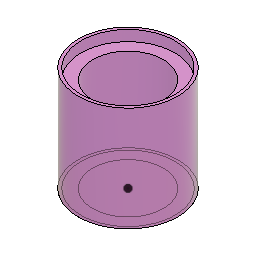
3_8 inch X-axis Bushing Holder v22 (Autodesk Fusion 360 design; units mm, degrees)
Autodesk Fusion 360 part; units mm, degrees
note: some values were not read from the file. Set by a fixed rule: which sketch regions a step uses.
sketch "Sketch1" plane through (0, 0, 0) normal (0, 0, 1) x (1, 0, 0) in component "Holder V1"
  circle A0 centre (0, 0) radius 6.325
  line L0 (0, 0) -> (-10.0178, 0) construction
  line L1 (-10.0178, -2.5) -> (-10.0178, 2.5) construction
  line L2 (-10.0178, 2.5) -> (-15.0178, 2.5)
  line L3 (-15.0178, 2.5) -> (-15.0178, -2.5)
  line L4 (-15.0178, -2.5) -> (-10.0178, -2.5)
  arc A1 (-10.0178, 2.5) -> (-10.0178, -2.5) centre (0, 0) ccw construction
  line L5 (-2.5, -10.0178) -> (-2.5, -15.0178)
  line L6 (-2.5, -15.0178) -> (2.5, -15.0178)
  line L7 (2.5, -15.0178) -> (2.5, -10.0178)
  line L8 (10.0178, -2.5) -> (15.0178, -2.5)
  line L9 (15.0178, -2.5) -> (15.0178, 2.5)
  line L10 (15.0178, 2.5) -> (10.0178, 2.5)
  line L11 (2.5, 10.0178) -> (2.5, 15.0178)
  line L12 (2.5, 15.0178) -> (-2.5, 15.0178)
  line L13 (-2.5, 15.0178) -> (-2.5, 10.0178)
  arc A2 (-10.0178, -2.5) -> (-2.5, -10.0178) centre (0, 0) ccw
  arc A3 (-2.5, -10.0178) -> (2.5, -10.0178) centre (0, 0) ccw construction
  arc A4 (2.5, -10.0178) -> (10.0178, -2.5) centre (0, 0) ccw
  arc A5 (10.0178, -2.5) -> (10.0178, 2.5) centre (0, 0) ccw construction
  arc A6 (10.0178, 2.5) -> (2.5, 10.0178) centre (0, 0) ccw
  arc A7 (-2.5, 10.0178) -> (-10.0178, 2.5) centre (0, 0) ccw
  arc A8 (2.5, 10.0178) -> (-2.5, 10.0178) centre (0, 0) ccw construction
  dimension "d13" = 12.65
  dimension "d14" = 5
  dimension "d15" = 20.65
  dimension "d17" = 360
  measures "d13" diameter of A0
  measures "d15" diameter of A2
extrude "Extrude1" add sketch "Sketch1" along normal blind 15.8 makes body 1 in component "Holder V1"
chamfer "Chamfer1" distance 1 angle 60 1 edges at (-5.897, 2.2872, 15.8) measured on face at (0.8333, -13.3511, 15.8) on bodies 1 in component "Holder V1"
sketch "Sketch1 (2)" plane through (0, 0, 0) normal (0, 0, 1) x (1, 0, 0) in component "Holder V2.3"
  arc A0 (-2.5, 10.0178) -> (-10.0178, 2.5) centre (0, 0) ccw construction
  line L0 (-10.0178, 2.5) -> (-15.0178, 2.5)
  line L1 (-15.0178, 2.5) -> (-15.0178, -2.5)
  line L2 (-15.0178, -2.5) -> (-10.0178, -2.5)
  arc A1 (-10.0178, -2.5) -> (-2.5, -10.0178) centre (0, 0) ccw
  line L3 (-2.5, -10.0178) -> (-2.5, -15.0178)
  line L4 (-2.5, -15.0178) -> (2.5, -15.0178)
  line L5 (2.5, -15.0178) -> (2.5, -10.0178)
  arc A2 (2.5, -10.0178) -> (10.0178, -2.5) centre (0, 0) ccw
  line L6 (10.0178, -2.5) -> (15.0178, -2.5)
  line L7 (15.0178, -2.5) -> (15.0178, 2.5)
  line L8 (15.0178, 2.5) -> (10.0178, 2.5)
  arc A3 (10.0178, 2.5) -> (2.5, 10.0178) centre (0, 0) ccw
  line L9 (2.5, 10.0178) -> (2.5, 15.0178)
  line L10 (2.5, 15.0178) -> (-2.5, 15.0178)
  line L11 (-2.5, 15.0178) -> (-2.5, 10.0178)
  circle A4 centre (0, 0) radius 7.325 construction
  line L12 (-14.0178, 1.5) -> (-14.0178, -1.5)
  line L13 (-14.0178, -1.5) -> (-9.2036, -1.5)
  arc A5 (-9.2036, -1.5) -> (-1.5, -9.2036) centre (0, 0) ccw
  line L14 (-1.5, -9.2036) -> (-1.5, -14.0178)
  line L15 (-1.5, -14.0178) -> (1.5, -14.0178)
  line L16 (1.5, -14.0178) -> (1.5, -9.2036)
  arc A6 (1.5, -9.2036) -> (9.2036, -1.5) centre (0, 0) ccw
  line L17 (9.2036, -1.5) -> (14.0178, -1.5)
  line L18 (14.0178, -1.5) -> (14.0178, 1.5)
  line L19 (14.0178, 1.5) -> (9.2036, 1.5)
  arc A7 (9.2036, 1.5) -> (1.5, 9.2036) centre (0, 0) ccw
  line L20 (1.5, 9.2036) -> (1.5, 14.0178)
  line L21 (1.5, 14.0178) -> (-1.5, 14.0178)
  line L22 (-1.5, 14.0178) -> (-1.5, 9.2036)
  arc A8 (-1.5, 9.2036) -> (-9.2036, 1.5) centre (0, 0) ccw
  line L23 (-9.2036, 1.5) -> (-14.0178, 1.5)
  circle A9 centre (0, 0) radius 6.325 construction
  circle A10 centre (0, 0) radius 6.3251
  dimension "d22" = 1
  dimension "d28" = 0.0001
  measures "d22" distance of L1
extrude "Extrude1'" add sketch "Sketch1 (2)" along normal blind 20 separate body makes body 2 in component "Holder V2.3"
sketch "Sketch1 (3)" plane through (0, 0, 0) normal (0, 0, 1) x (1, 0, 0) in component "Holder V3.1"
  circle A0 centre (0, 0) radius 5
  circle A1 centre (0, 0) radius 6.4 construction
  line L0 (0, 0) -> (-9.4, 0) construction
  line L1 (-9.1848, 0) -> (-9.1848, 2) construction
  line L2 (-9.1848, 2) -> (-17.1959, 2)
  line L3 (-17.1959, 2) -> (-17.1959, -2)
  line L4 (-17.1959, -2) -> (-9.1848, -2)
  line L5 (-9.1848, -2) -> (-9.1848, 0) construction
  arc A2 (-9.4, 0) -> (-9.1848, -2) centre (0, 0) ccw construction
  arc A3 (-9.1848, 2) -> (-9.4, 0) centre (0, 0) ccw construction
  line L6 (-2, -9.1848) -> (-2, -17.1959)
  line L7 (-2, -17.1959) -> (2, -17.1959)
  line L8 (2, -17.1959) -> (2, -9.1848)
  line L9 (9.1848, -2) -> (17.1959, -2)
  line L10 (17.1959, -2) -> (17.1959, 2)
  line L11 (17.1959, 2) -> (9.1848, 2)
  line L12 (2, 9.1848) -> (2, 17.1959)
  line L13 (2, 17.1959) -> (-2, 17.1959)
  line L14 (-2, 17.1959) -> (-2, 9.1848)
  arc A4 (9.1848, -2) -> (9.1848, 2) centre (0, 0) ccw construction
  arc A5 (9.1848, 2) -> (2, 9.1848) centre (0, 0) ccw
  arc A6 (-2, 9.1848) -> (-9.1848, 2) centre (0, 0) ccw
  arc A7 (-9.1848, -2) -> (-2, -9.1848) centre (0, 0) ccw
  arc A8 (2, -9.1848) -> (9.1848, -2) centre (0, 0) ccw
  arc A9 (-2, -9.1848) -> (2, -9.1848) centre (0, 0) ccw construction
  arc A10 (2, 9.1848) -> (-2, 9.1848) centre (0, 0) ccw construction
  dimension "d29" = 18.8
  dimension "d30" = 12.8
  dimension "d31" = 10
  dimension "d32" = 4
  dimension "d34" = 360
  measures "d29" diameter of A7
  measures "d30" diameter of A1
  measures "d31" diameter of A0
extrude "Extrude1''" add sketch "Sketch1 (3)" along normal blind 16 separate body makes body 3 in component "Holder V3.1"
chamfer "Chamfer1'" distance 1 angle 45 1 edges at (-4.6616, 1.8081, 16) on bodies 3 in component "Holder V3.1"
fillet "Fillet1" radius 1.5 32 edges at (6.6468, 6.6468, 16) (2, 13.1903, 16) (0, 17.1959, 16) (-2, 13.1903, 16) (-6.6468, 6.6468, 16) (-13.1903, 2, 16) (-17.1959, 0, 16) (-13.1903, -2, 16) (-6.6468, -6.6468, 16) (-2, -13.1903, 16) (0, -17.1959, 16) (2, -13.1903, 16) (6.6468, -6.6468, 16) (13.1903, -2, 16) (17.1959, 0, 16) (13.1903, 2, 16) (17.1959, 0, 0) (13.1903, 2, 0) (6.6468, 6.6468, 0) (2, 13.1903, 0) (-2, 13.1903, 0) (0, 17.1959, 0) (-6.6468, 6.6468, 0) (-13.1903, 2, 0) (-17.1959, 0, 0) (-13.1903, -2, 0) (-2, -13.1903, 0) (0, -17.1959, 0) (2, -13.1903, 0) (6.6468, -6.6468, 0) (13.1903, -2, 0) (-6.6468, -6.6468, 0) on bodies 3 in component "Holder V3.1"
sketch "Sketch1 (4)" plane through (0, 0, 0) normal (0, 1, 0) x (1, 0, 0) in component "Holder Test V4.2"
  circle A0 centre (0, 0) radius 6.3
  circle A1 centre (0, 0) radius 7.8
  circle A2 centre (16, 0) radius 6.4
  circle A3 centre (16, 0) radius 7.9
  circle A4 centre (32, 0) radius 6.5
  circle A5 centre (32, 0) radius 8
  circle A6 centre (0, 16) radius 6.8
  circle A7 centre (0, 16) radius 8.3
  circle A8 centre (16, 16) radius 6.7
  circle A9 centre (16, 16) radius 8.2
  circle A10 centre (32, 16) radius 6.6
  circle A11 centre (32, 16) radius 8.1
  line L0 (-0.5169, -7.65) -> (0.3, -7.65) construction
  line L1 (0.3, -7.65) -> (0.3, -5.9) construction
  line L2 (0.3, -5.9) -> (-0.5169, -5.9) construction
  line L3 (-0.5169, -5.9) -> (-0.5169, -7.65) construction
  line L4 (15.5931, -7.9846) -> (16.0546, -7.9846) construction
  line L5 (16.0546, -7.9846) -> (16.0546, -6.2346) construction
  line L6 (16.0546, -6.2346) -> (15.5931, -6.2346) construction
  line L7 (15.5931, -6.2346) -> (15.5931, -7.9846) construction
  line L8 (31.4703, -7.85) -> (32.3, -7.85) construction
  line L9 (32.3, -7.85) -> (32.3, -6.1) construction
  line L10 (32.3, -6.1) -> (31.4703, -6.1) construction
  line L11 (31.4703, -6.1) -> (31.4703, -7.85) construction
  line L12 (31.4797, 22.7) -> (32.3, 22.7) construction
  line L13 (32.3, 22.7) -> (32.3, 24.45) construction
  line L14 (32.3, 24.45) -> (31.4797, 24.45) construction
  line L15 (31.4797, 24.45) -> (31.4797, 22.7) construction
  line L16 (15.3335, 22.8) -> (16.2, 22.8) construction
  line L17 (16.2, 22.8) -> (16.2, 24.55) construction
  line L18 (16.2, 24.55) -> (15.3335, 24.55) construction
  line L19 (15.3335, 24.55) -> (15.3335, 22.8) construction
  line L20 (-0.6, 22.9) -> (0.2306, 22.9) construction
  line L21 (0.2306, 22.9) -> (0.2306, 24.65) construction
  line L22 (0.2306, 24.65) -> (-0.6, 24.65) construction
  line L23 (-0.6, 24.65) -> (-0.6, 22.9) construction
  line L24 (0, 0) -> (32, 0)
  line L25 (32, 0) -> (32, 16)
  line L26 (32, 16) -> (0, 16)
  line L27 (0, 16) -> (0, 0)
  line L28 (0, 16) -> (0, 17.5)
  line L29 (0, 17.5) -> (32, 17.5)
  line L30 (32, 17.5) -> (32, 16)
  line L31 (32, 0) -> (32, -1.5)
  line L32 (32, -1.5) -> (0, -1.5)
  line L33 (0, -1.5) -> (0, 0)
  line L34 (0, -1.5) -> (-1.5, -1.5)
  line L35 (-1.5, -1.5) -> (-1.5, 17.5)
  line L36 (-1.5, 17.5) -> (0, 17.5)
  line L37 (32, 17.5) -> (33.5, 17.5)
  line L38 (33.5, 17.5) -> (33.5, -1.5)
  line L39 (33.5, -1.5) -> (32, -1.5)
  line L40 (-1.5, 0) -> (32, 17.5)
  line L41 (0, -1.5) -> (33.5, 16)
  line L42 (32, 0) -> (33.5, 0)
  line L43 (33.5, 0) -> (0, 17.5)
  line L44 (32, -1.5) -> (-1.5, 16)
  line L45 (-1.5, 0) -> (-7.8, 0) construction
  line L46 (-7.8, 0) -> (-10.3, 0)
  line L47 (-10.3, 0) -> (-10.3, -2.5)
  line L48 (-10.3, -2.5) -> (-7.3885, -2.5)
  dimension "d40" = 12.6
  dimension "d41" = 15.6
  dimension "d46" = 12.8
  dimension "d47" = 13
  dimension "d48" = 13.2
  dimension "d49" = 13.4
  dimension "d50" = 13.6
  dimension "d51" = 15.8
  dimension "d52" = 16
  dimension "d53" = 16.2
  dimension "d54" = 16.4
  dimension "d55" = 16.6
  dimension "d61" = 2.5
  dimension "d62" = 2.5
  measures "d40" diameter of A0
  measures "d41" diameter of A1
  measures "d46" diameter of A2
  measures "d47" diameter of A4
  measures "d48" diameter of A10
  measures "d49" diameter of A8
  measures "d50" diameter of A6
  measures "d51" diameter of A3
  measures "d52" diameter of A5
  measures "d53" diameter of A11
  measures "d54" diameter of A9
  measures "d55" diameter of A7
extrude "Extrude1'''" add sketch "Sketch1 (4)" along normal blind 5 separate body contours A0 A1 L24 L32 | A0 A1 L24 L41 | A0 A1 L40 L41 | A0 A1 L32 L35 | A1 A3 L24 L32 | A0 A1 A7 L27 L40 | A1 A3 L40 L41 L44 | A0 A1 A7 L27 L35 | A2 A3 L24 L32 | A2 A3 L24 L41 | A2 A3 L41 L44 | A1 A7 L35 | A1 L46 L47 L48 | A2 A3 L32 | A1 A7 L27 | A1 A7 L27 | A1 A6 A7 L27 L44 | A9 L40 L44 | A3 A9 L40 L44 | A3 A9 L41 L44 | A1 A6 A7 L27 L35 | A6 A7 A9 L29 L35 | A2 A3 L24 L32 | A3 A5 L24 L32 | A2 A3 L24 L44 | A6 A7 L43 L44 | A7 A9 L43 L44 | A3 A9 L40 L43 | A8 A9 L40 L43 L44 | A9 L44 | A3 A9 | A2 L41 L44 | A2 A3 L41 L44 | A7 A8 A9 A11 L29 | A7 A9 L29 | A4 A5 L32 L38 | A4 A5 L24 L32 | A6 A7 A9 L26 L43 | A8 L40 L43 | A8 A9 L40 L41 L43 | A3 A9 L41 L43 | A3 A5 L41 L43 L44 | A7 A8 L26 L29 | A7 A9 L26 L29 | A9 A10 A11 L29 L38 | A9 A11 L29 | A6 A9 L26 L29 | A4 A5 L24 L44 | A7 A9 L26 | A7 A8 A9 L26 L43 | A9 L41 L43 | A9 A10 L26 L29 | A9 A11 L26 L29 | A8 A11 L26 L29 | A4 A5 L43 L44 | A4 A5 A11 L25 L38 | A5 A11 L38 | A8 A9 A11 L26 L40 | A9 L41 | A4 A5 A11 L25 L43 | A9 A10 A11 L26 L40 | A9 A11 L26 | A5 A10 A11 L25 L38 | A5 A11 L25 | A9 A11 L40 L41 | A5 A10 A11 L25 L41 | A5 A11 L25 | A10 A11 L40 L41 makes body 4 in component "Holder Test V4.2"
sketch "Sketch1 (5)" plane through (0, 0, 0) normal (0, 1, 0) x (1, 0, 0) in component "Holder V4.2"
  circle A0 centre (0, 0) radius 6.7
  circle A1 centre (0, 0) radius 9.45
  dimension "d63" = 13.4
  dimension "d64" = 18.9
  measures "d63" diameter of A0
  measures "d64" diameter of A1
extrude "Extrude1''''" add sketch "Sketch1 (5)" along normal blind 16 separate body makes body 5 in component "Holder V4.2"
sketch "Sketch1 (6)" plane through (0, 0, 0) normal (0, 1, 0) x (1, 0, 0) in component "Holder (for bronze 1/2in OD bushings) V5"
  circle A0 centre (0, 0) radius 6.65
  circle A1 centre (0, 0) radius 9.4
  circle A2 centre (0, 0) radius 8.8562
  dimension "d63_1" = 13.3
  dimension "d64_1" = 18.8
  dimension "d67" = 17.7125
  measures "d63_1" diameter of A0
  measures "d64_1" diameter of A1
  measures "d67" diameter of A2
extrude "Extrude1'''''" add sketch "Sketch1 (6)" along normal blind 17.8 separate body contours A1 | A2 makes body 6 in component "Holder (for bronze 1/2in OD bushings) V5"
extrude "Extrude2" add sketch "Sketch1 (6)" along normal blind 2 from surface at 17.8 contours A1 bodies 6 in component "Holder (for bronze 1/2in OD bushings) V5"
component "Holder V1" placed x (1, 0, 0) y (0, 1, 0) z (0, 0, 1) at (0, 0, 0)
component "Holder V2.3" placed x (1, 0, 0) y (0, 1, 0) z (0, 0, 1) at (0, 0, 0)
component "Holder V3.1" placed x (1, 0, 0) y (0, 1, 0) z (0, 0, 1) at (0, 0, 0)
component "Holder Test V4.2" placed x (1, 0, 0) y (0, 1, 0) z (0, 0, 1) at (0, 0, 0)
component "Holder V4.2" placed x (1, 0, 0) y (0, 1, 0) z (0, 0, 1) at (0, 0, 0)
component "Holder (for bronze 1/2in OD bushings) V5" placed x (1, 0, 0) y (0, 1, 0) z (0, 0, 1) at (0, 0, 0)
equation "d15 = d13 + ( ( 2 * 4 ) * 1 mm )"
equation "d29 = d30 + ( ( 3 * 2 ) * 1 mm )"
equation "d41 = d40 + 3 mm"
equation "d46 = d40 + 0.2 mm"
equation "d47 = d46 + 0.2 mm"
equation "d48 = d47 + 0.2 mm"
equation "d49 = d48 + 0.2 mm"
equation "d50 = d49 + 0.2 mm"
equation "d51 = d46 + 3 mm"
equation "d52 = d47 + 3 mm"
equation "d53 = d48 + 3 mm"
equation "d54 = d49 + 3 mm"
equation "d55 = d50 + 3 mm"
equation "d62 = d61"
equation "d64 = d63 + ( 2 * 2.75 ) * 1 mm"
equation "d64_1 = d63_1 + ( 2 * 2.75 ) * 1 mm"
equation "d67 = ( 11 / 16 * 25.4 ) * 1 mm + 0.25 mm"
